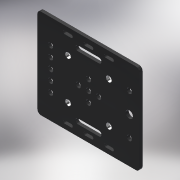
# Autodesk Inventor part: 20mm gantry plate
Saved by Autodesk Inventor 2020.3 (Build 243373000, 373)
## iProperties
Created: 2016-04-10
Part Number: 20mm gantry plate
Material: Aluminum 6061
Document SubType Name: Modeling
Designer: Ben
Density: 2.7 g/cm^3
Appearance: Aluminum - Flat
Author: Ben
Autodesk Inventor part; units mm, degrees
ref_plane "YZ Plane" through (0, 0, 0) normal (1, 0, 0) x (0, 1, 0)
ref_plane "XZ Plane" through (0, 0, 0) normal (0, 1, 0) x (-1, 0, 0)
ref_plane "XY Plane" through (0, 0, 0) normal (0, 0, 1) x (1, 0, 0)
sketch "Sketch1" plane through (0, 0, 0) normal (0, 0, 1) x (1, 0, 0)
  line L0 (-50, 44) -> (50, 44)
  line L1 (50, 44) -> (50, -44)
  line L2 (50, -44) -> (-50, -44)
  line L3 (-50, -44) -> (-50, 44)
  line L4 (0, 44) -> (0, -44) construction
  line L5 (-50, 0) -> (50, 0) construction
  point P0 (0, 0)
  dimension "d0" = 100
  dimension "d1" = 88
  constraints: 12 end point, 6 midpoint, 2 parallel, 1 horizontal, 1 perpendicular
  measures "d0" distance of L1.end L2.end
  measures "d1" distance of L0.end L1.end
extrude "Extrusion1" add sketch "Sketch1" along normal blind 3
sketch "Sketch2" plane through (0, 0, 3) normal (0, 0, 1) x (1, 0, 0)
  line L0 (-50, 44) -> (-50, -44) projected
  line L1 (50, -44) -> (50, 44) projected
  circle A0 centre (0, 0) radius 2.5
  circle A1 centre (0, 10) radius 2.5
  line L2 (0, 0) -> (0, 20.5611) construction
  circle A2 centre (-10, 0) radius 2.5
  circle A3 centre (0, -10) radius 2.5
  circle A4 centre (10, 0) radius 2.5
  circle A5 centre (-37.1, 0) radius 2.5
  circle A6 centre (-37.1, -10) radius 2.5
  circle A7 centre (-37.1, -20) radius 2.5
  circle A8 centre (-37.1, 10) radius 2.5
  circle A9 centre (-37.1, 0) radius 2.5
  circle A10 centre (-37.1, -10) radius 2.5
  circle A11 centre (-37.1, 20) radius 2.5
  circle A12 centre (-37.1, 10) radius 2.5
  circle A13 centre (-37.1, 0) radius 2.5
  line L3 (0, 0) -> (-50, 0) construction
  circle A14 centre (40, 0) radius 3.6 construction
  circle A15 centre (40, 20) radius 3.6 construction
  circle A16 centre (40, -20) radius 3.6 construction
  circle A17 centre (40, 0) radius 3.6 construction
  circle A18 centre (40, 0) radius 3.6
  line L4 (40, 0) -> (40, 20) construction
  line L5 (40, 0) -> (40, -20) construction
  circle A19 centre (40, 20) radius 2.5
  circle A20 centre (40, -20) radius 2.5
  dimension "d4" = 5
  dimension "d5" = 5
  dimension "d6" = 10
  dimension "d9" = 360
  dimension "d11" = 5
  dimension "d12" = 12.9
  dimension "d15" = 10
  dimension "d18" = 10
  dimension "d28" = 20
  dimension "d31" = 20
  dimension "d64" = 7.2
  dimension "d65" = 5
  dimension "d66" = 5
  constraints: 21 centre point, 8 end point, 6 vertical, 4 coincident, 2 point on line, 1 midpoint, 1 parallel, 31 other
  measures "d4" diameter of A0
  measures "d5" diameter of A1
  measures "d6" distance of L2.start A1.centre
  measures "d11" diameter of A5
  measures "d12" distance from line of A5.centre L0
  measures "d15" distance of A5.centre A6.centre
  measures "d18" distance of A5.centre A8.centre
  measures "d28" distance of A14.centre L4.end
  measures "d31" distance of A14.centre L5.end
  measures "d64" diameter of A18
  measures "d65" diameter of A19
  measures "d66" diameter of A20
extrude "Extrusion2" cut sketch "Sketch2" against normal up to next
sketch "Sketch3" plane through (0, 0, 3) normal (0, 0, 1) x (1, 0, 0)
  circle A0 centre (0, 0) radius 2.5 projected
  line L0 (50, 44) -> (-50, 44) projected
  line L1 (-50, -44) -> (50, -44) projected
  line L2 (0, 0) -> (0, -39.6664) construction
  line L3 (0, 0) -> (-44.4767, 0) construction
  line L4 (-3.25, -38) -> (3.25, -38) construction
  line L5 (-3.25, -39.5) -> (3.25, -39.5)
  line L6 (3.25, -36.5) -> (-3.25, -36.5)
  arc A1 (-3.25, -36.5) -> (-3.25, -39.5) centre (-3.25, -38) ccw
  arc A2 (3.25, -39.5) -> (3.25, -36.5) centre (3.25, -38) ccw
  line L7 (16.9, -38) -> (23.4, -38) construction
  line L8 (16.9, -39.5) -> (23.4, -39.5)
  line L9 (23.4, -36.5) -> (16.9, -36.5)
  arc A3 (16.9, -36.5) -> (16.9, -39.5) centre (16.9, -38) ccw
  arc A4 (23.4, -39.5) -> (23.4, -36.5) centre (23.4, -38) ccw
  line L10 (-23.4, -38) -> (-16.9, -38) construction
  line L11 (-23.4, -39.5) -> (-16.9, -39.5)
  line L12 (-16.9, -36.5) -> (-23.4, -36.5)
  arc A5 (-23.4, -36.5) -> (-23.4, -39.5) centre (-23.4, -38) ccw
  arc A6 (-16.9, -39.5) -> (-16.9, -36.5) centre (-16.9, -38) ccw
  line L13 (-3.25, -38) -> (3.25, -38) construction
  line L14 (-3.25, -39.5) -> (3.25, -39.5)
  line L15 (3.25, -36.5) -> (-3.25, -36.5)
  arc A7 (-3.25, -36.5) -> (-3.25, -39.5) centre (-3.25, -38) ccw
  arc A8 (3.25, -39.5) -> (3.25, -36.5) centre (3.25, -38) ccw
  line L16 (-3.25, 38) -> (3.25, 38) construction
  line L17 (-3.25, 39.5) -> (3.25, 39.5)
  line L18 (3.25, 36.5) -> (-3.25, 36.5)
  arc A9 (-3.25, 39.5) -> (-3.25, 36.5) centre (-3.25, 38) ccw
  arc A10 (3.25, 36.5) -> (3.25, 39.5) centre (3.25, 38) ccw
  arc A11 (16.9, 39.5) -> (16.9, 36.5) centre (16.9, 38) ccw
  line L19 (23.4, 36.5) -> (16.9, 36.5)
  line L20 (16.9, 38) -> (23.4, 38) construction
  line L21 (16.9, 39.5) -> (23.4, 39.5)
  arc A12 (23.4, 36.5) -> (23.4, 39.5) centre (23.4, 38) ccw
  arc A13 (-23.4, 39.5) -> (-23.4, 36.5) centre (-23.4, 38) ccw
  line L22 (-16.9, 36.5) -> (-23.4, 36.5)
  line L23 (-23.4, 38) -> (-16.9, 38) construction
  line L24 (-23.4, 39.5) -> (-16.9, 39.5)
  arc A14 (-16.9, 36.5) -> (-16.9, 39.5) centre (-16.9, 38) ccw
  arc A15 (-3.25, 39.5) -> (-3.25, 36.5) centre (-3.25, 38) ccw
  line L25 (3.25, 36.5) -> (-3.25, 36.5)
  line L26 (-3.25, 38) -> (3.25, 38) construction
  line L27 (-3.25, 39.5) -> (3.25, 39.5)
  arc A16 (3.25, 36.5) -> (3.25, 39.5) centre (3.25, 38) ccw
  line L28 (50, -44) -> (-50, -44) projected
  line L29 (0, -44) -> (0, -31) construction
  line L30 (-10.32, -31) -> (10.32, -31) construction
  line L31 (-10.32, -33.5) -> (10.32, -33.5)
  line L32 (10.32, -28.5) -> (-10.32, -28.5)
  arc A17 (-10.32, -28.5) -> (-10.32, -33.5) centre (-10.32, -31) ccw
  arc A18 (10.32, -33.5) -> (10.32, -28.5) centre (10.32, -31) ccw
  line L33 (-10.32, 33.5) -> (10.32, 33.5)
  line L34 (10.32, 28.5) -> (-10.32, 28.5)
  arc A19 (-10.32, 33.5) -> (-10.32, 28.5) centre (-10.32, 31) ccw
  line L35 (0, 44) -> (0, 31) construction
  line L36 (-10.32, 31) -> (10.32, 31) construction
  line L37 (-10.32, 33.5) -> (10.32, 33.5)
  line L38 (10.32, 28.5) -> (-10.32, 28.5)
  arc A20 (-10.32, 33.5) -> (-10.32, 28.5) centre (-10.32, 31) ccw
  arc A21 (10.32, 28.5) -> (10.32, 33.5) centre (10.32, 31) ccw
  point P0 (0, -38)
  point P1 (20.15, -38)
  point P2 (-20.15, -38)
  point P3 (0, -38)
  point P4 (0, 38)
  point P5 (20.15, 38)
  point P6 (-20.15, 38)
  point P7 (0, 38)
  dimension "d38" = 3
  dimension "d40" = 6.5
  dimension "d43" = 20.15
  dimension "d46" = 20.15
  dimension "d59" = 6
  dimension "d61" = 13
  dimension "d62" = 10.32
  dimension "d63" = 5
  constraints: 92 end point, 42 point on circle, 37 symmetric about line, 21 centre point, 8 tangent, 3 horizontal, 3 midpoint, 3 parallel, 2 point on line, 1 perpendicular, 47 other
  measures "d38" diameter of A2
  measures "d40" distance of L4.end L4.start
  measures "d43" distance of L6.end L9.end
  measures "d46" distance of L6.end L12.end
  measures "d59" distance from line of L1 point (0, -38)
  measures "d61" distance of L29.start L29.end
  measures "d62" distance of L29.end L30.end
  measures "d63" diameter of A18
extrude "Extrusion3" cut sketch "Sketch3" against normal up to next contours A1 L6 A2 L5 | A3 L9 A4 L8 | A5 L12 A6 L11 | L17 A10 L18 A9 | L21 A12 L19 A11 | L24 A14 L22 A13 | A17 L32 A18 L31 | L33 A21 L34 A19
fillet "Fillet1" radius 3.38 4 edges at (50, -44, 1.5) (50, 44, 1.5) (-50, -44, 1.5) (-50, 44, 1.5)
sketch "Sketch5" plane through (0, 0, 3) normal (0, 0, 1) x (1, 0, 0)
  line L0 (-20, 20) -> (20, 20) construction
  line L1 (20, 20) -> (20, -20) construction
  line L2 (20, -20) -> (-20, -20) construction
  line L3 (-20, -20) -> (-20, 20) construction
  circle A0 centre (0, 0) radius 2.5 projected
  line L4 (-20, 20) -> (20, -20) construction
  line L5 (20, 20) -> (-20, -20) construction
  circle A1 centre (-20, 20) radius 2.75
  circle A2 centre (20, 20) radius 2.75
  circle A3 centre (-20, -20) radius 2.75
  circle A4 centre (20, -20) radius 2.75
  dimension "d67" = 40
  dimension "d68" = 40
  dimension "d69" = 5.5
  dimension "d70" = 5.5
  dimension "d71" = 5.5
  dimension "d72" = 5.5
  constraints: 12 end point, 4 centre point, 4 coincident, 2 midpoint, 2 parallel, 1 horizontal, 1 perpendicular
  measures "d67" distance of L1.end L2.end
  measures "d68" distance of L0.end L1.end
  measures "d69" diameter of A1
  measures "d70" diameter of A2
  measures "d71" diameter of A3
  measures "d72" diameter of A4
extrude "Extrusion5" cut sketch "Sketch5" against normal through all contours A1 | A2 | A3 | A4
body "Solid1"
